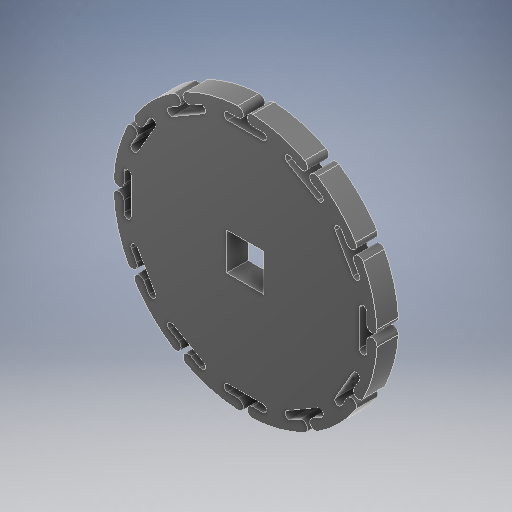
# Autodesk Inventor part: Sprocket
Saved by Autodesk Inventor 2026.1 (Build 301233000, 233)
## iProperties
Created: 2025-10-04
Part Number: Sprocket
Material: Plastic, Opaque Black
Document SubType Name: Modeling
Designer: Teddy
Density: 0.952 g/cm^3
Appearance: Smooth - Black
Author: Teddy
Autodesk Inventor part; units mm, degrees
ref_plane "YZ Plane" through (0, 0, 0) normal (1, 0, 0) x (0, 1, 0)
ref_plane "XZ Plane" through (0, 0, 0) normal (0, 1, 0) x (-1, 0, 0)
ref_plane "XY Plane" through (0, 0, 0) normal (0, 0, 1) x (1, 0, 0)
sketch "Sketch1" plane through (0, 0, 0) normal (0, 0, 1) x (1, 0, 0)
  arc A0 (-1.3226, 23.4577) -> (-10.5835, 20.9763) centre (0, 0) ccw
  line L0 (-3.302, -3.302) -> (3.302, -3.302)
  line L1 (3.302, -3.302) -> (3.302, 3.302)
  line L2 (3.302, 3.302) -> (-3.302, 3.302)
  line L3 (-3.302, 3.302) -> (-3.302, -3.302)
  line L4 (-3.302, -3.302) -> (3.302, 3.302) construction
  line L5 (3.302, -3.302) -> (-3.302, 3.302) construction
  line L6 (0, 0) -> (0, 9.525) construction
  line L7 (-3.175, 20.955) -> (3.175, 20.955)
  line L8 (-3.175, 20.32) -> (3.175, 20.32)
  arc A1 (-3.175, 21.59) -> (-3.175, 20.32) centre (-3.175, 20.955) ccw
  arc A2 (3.175, 20.32) -> (3.175, 21.59) centre (3.175, 20.955) ccw
  arc A3 (-1.27, 21.59) -> (-1.3226, 23.4577) centre (-1.27, 22.5246) ccw
  arc A4 (1.3226, 23.4577) -> (1.27, 21.59) centre (1.27, 22.5246) ccw
  line L9 (-1.27, 22.5246) -> (1.27, 22.5246) construction
  line L10 (3.175, 21.59) -> (1.27, 21.59)
  line L11 (-1.27, 21.59) -> (-3.175, 21.59)
  arc A5 (-13.5446, 17.11) -> (-12.9096, 16.0101) centre (-13.2271, 16.5601) ccw
  line L12 (-12.9096, 16.0101) -> (-7.4104, 19.1851)
  arc A6 (-7.4104, 19.1851) -> (-8.0454, 20.285) centre (-7.7279, 19.7351) ccw
  arc A7 (-10.5835, 20.9763) -> (-9.6951, 19.3325) centre (-10.1625, 20.1419) ccw
  line L13 (-8.0454, 20.285) -> (-9.6951, 19.3325)
  line L14 (-11.8949, 18.0625) -> (-13.5446, 17.11)
  arc A8 (-11.8949, 18.0625) -> (-12.8743, 19.6537) centre (-12.3622, 18.8719) ccw
  arc A9 (-20.285, 8.0454) -> (-19.1851, 7.4104) centre (-19.7351, 7.7279) ccw
  line L15 (-19.1851, 7.4104) -> (-16.0101, 12.9096)
  arc A10 (-16.0101, 12.9096) -> (-17.11, 13.5446) centre (-16.5601, 13.2271) ccw
  arc A11 (-19.6537, 12.8743) -> (-18.0625, 11.8949) centre (-18.8719, 12.3622) ccw
  line L16 (-17.11, 13.5446) -> (-18.0625, 11.8949)
  line L17 (-19.3325, 9.6951) -> (-20.285, 8.0454)
  arc A12 (-19.3325, 9.6951) -> (-20.9763, 10.5835) centre (-20.1419, 10.1625) ccw
  arc A13 (-21.59, -3.175) -> (-20.32, -3.175) centre (-20.955, -3.175) ccw
  line L18 (-20.32, -3.175) -> (-20.32, 3.175)
  arc A14 (-20.32, 3.175) -> (-21.59, 3.175) centre (-20.955, 3.175) ccw
  arc A15 (-23.4577, 1.3226) -> (-21.59, 1.27) centre (-22.5246, 1.27) ccw
  line L19 (-21.59, 3.175) -> (-21.59, 1.27)
  line L20 (-21.59, -1.27) -> (-21.59, -3.175)
  arc A16 (-21.59, -1.27) -> (-23.4577, -1.3226) centre (-22.5246, -1.27) ccw
  arc A17 (-17.11, -13.5446) -> (-16.0101, -12.9096) centre (-16.5601, -13.2271) ccw
  line L21 (-16.0101, -12.9096) -> (-19.1851, -7.4104)
  arc A18 (-19.1851, -7.4104) -> (-20.285, -8.0454) centre (-19.7351, -7.7279) ccw
  arc A19 (-20.9763, -10.5835) -> (-19.3325, -9.6951) centre (-20.1419, -10.1625) ccw
  line L22 (-20.285, -8.0454) -> (-19.3325, -9.6951)
  line L23 (-18.0625, -11.8949) -> (-17.11, -13.5446)
  arc A20 (-18.0625, -11.8949) -> (-19.6537, -12.8743) centre (-18.8719, -12.3622) ccw
  arc A21 (-8.0454, -20.285) -> (-7.4104, -19.1851) centre (-7.7279, -19.7351) ccw
  line L24 (-7.4104, -19.1851) -> (-12.9096, -16.0101)
  arc A22 (-12.9096, -16.0101) -> (-13.5446, -17.11) centre (-13.2271, -16.5601) ccw
  arc A23 (-12.8743, -19.6537) -> (-11.8949, -18.0625) centre (-12.3622, -18.8719) ccw
  line L25 (-13.5446, -17.11) -> (-11.8949, -18.0625)
  line L26 (-9.6951, -19.3325) -> (-8.0454, -20.285)
  arc A24 (-9.6951, -19.3325) -> (-10.5835, -20.9763) centre (-10.1625, -20.1419) ccw
  arc A25 (3.175, -21.59) -> (3.175, -20.32) centre (3.175, -20.955) ccw
  line L27 (3.175, -20.32) -> (-3.175, -20.32)
  arc A26 (-3.175, -20.32) -> (-3.175, -21.59) centre (-3.175, -20.955) ccw
  arc A27 (-1.3226, -23.4577) -> (-1.27, -21.59) centre (-1.27, -22.5246) ccw
  line L28 (-3.175, -21.59) -> (-1.27, -21.59)
  line L29 (1.27, -21.59) -> (3.175, -21.59)
  arc A28 (1.27, -21.59) -> (1.3226, -23.4577) centre (1.27, -22.5246) ccw
  arc A29 (13.5446, -17.11) -> (12.9096, -16.0101) centre (13.2271, -16.5601) ccw
  line L30 (12.9096, -16.0101) -> (7.4104, -19.1851)
  arc A30 (7.4104, -19.1851) -> (8.0454, -20.285) centre (7.7279, -19.7351) ccw
  arc A31 (10.5835, -20.9763) -> (9.6951, -19.3325) centre (10.1625, -20.1419) ccw
  line L31 (8.0454, -20.285) -> (9.6951, -19.3325)
  line L32 (11.8949, -18.0625) -> (13.5446, -17.11)
  arc A32 (11.8949, -18.0625) -> (12.8743, -19.6537) centre (12.3622, -18.8719) ccw
  arc A33 (20.285, -8.0454) -> (19.1851, -7.4104) centre (19.7351, -7.7279) ccw
  line L33 (19.1851, -7.4104) -> (16.0101, -12.9096)
  arc A34 (16.0101, -12.9096) -> (17.11, -13.5446) centre (16.5601, -13.2271) ccw
  arc A35 (19.6537, -12.8743) -> (18.0625, -11.8949) centre (18.8719, -12.3622) ccw
  line L34 (17.11, -13.5446) -> (18.0625, -11.8949)
  line L35 (19.3325, -9.6951) -> (20.285, -8.0454)
  arc A36 (19.3325, -9.6951) -> (20.9763, -10.5835) centre (20.1419, -10.1625) ccw
  arc A37 (21.59, 3.175) -> (20.32, 3.175) centre (20.955, 3.175) ccw
  line L36 (20.32, 3.175) -> (20.32, -3.175)
  arc A38 (20.32, -3.175) -> (21.59, -3.175) centre (20.955, -3.175) ccw
  arc A39 (23.4577, -1.3226) -> (21.59, -1.27) centre (22.5246, -1.27) ccw
  line L37 (21.59, -3.175) -> (21.59, -1.27)
  line L38 (21.59, 1.27) -> (21.59, 3.175)
  arc A40 (21.59, 1.27) -> (23.4577, 1.3226) centre (22.5246, 1.27) ccw
  arc A41 (17.11, 13.5446) -> (16.0101, 12.9096) centre (16.5601, 13.2271) ccw
  line L39 (16.0101, 12.9096) -> (19.1851, 7.4104)
  arc A42 (19.1851, 7.4104) -> (20.285, 8.0454) centre (19.7351, 7.7279) ccw
  arc A43 (20.9763, 10.5835) -> (19.3325, 9.6951) centre (20.1419, 10.1625) ccw
  line L40 (20.285, 8.0454) -> (19.3325, 9.6951)
  line L41 (18.0625, 11.8949) -> (17.11, 13.5446)
  arc A44 (18.0625, 11.8949) -> (19.6537, 12.8743) centre (18.8719, 12.3622) ccw
  arc A45 (8.0454, 20.285) -> (7.4104, 19.1851) centre (7.7279, 19.7351) ccw
  line L42 (7.4104, 19.1851) -> (12.9096, 16.0101)
  arc A46 (12.9096, 16.0101) -> (13.5446, 17.11) centre (13.2271, 16.5601) ccw
  arc A47 (12.8743, 19.6537) -> (11.8949, 18.0625) centre (12.3622, 18.8719) ccw
  line L43 (13.5446, 17.11) -> (11.8949, 18.0625)
  line L44 (9.6951, 19.3325) -> (8.0454, 20.285)
  arc A48 (9.6951, 19.3325) -> (10.5835, 20.9763) centre (10.1625, 20.1419) ccw
  arc A49 (-12.8743, 19.6537) -> (-19.6537, 12.8743) centre (0, 0) ccw
  arc A50 (-10.5835, 20.9763) -> (-12.8743, 19.6537) centre (0, 0) ccw construction
  arc A51 (10.5835, 20.9763) -> (1.3226, 23.4577) centre (0, 0) ccw
  arc A52 (12.8743, 19.6537) -> (10.5835, 20.9763) centre (0, 0) ccw construction
  arc A53 (19.6537, 12.8743) -> (12.8743, 19.6537) centre (0, 0) ccw
  arc A54 (20.9763, 10.5835) -> (19.6537, 12.8743) centre (0, 0) ccw construction
  arc A55 (23.4577, 1.3226) -> (20.9763, 10.5835) centre (0, 0) ccw
  arc A56 (23.4577, -1.3226) -> (23.4577, 1.3226) centre (0, 0) ccw construction
  arc A57 (20.9763, -10.5835) -> (23.4577, -1.3226) centre (0, 0) ccw
  arc A58 (19.6537, -12.8743) -> (20.9763, -10.5835) centre (0, 0) ccw construction
  arc A59 (12.8743, -19.6537) -> (19.6537, -12.8743) centre (0, 0) ccw
  arc A60 (10.5835, -20.9763) -> (12.8743, -19.6537) centre (0, 0) ccw construction
  arc A61 (1.3226, -23.4577) -> (10.5835, -20.9763) centre (0, 0) ccw
  arc A62 (-1.3226, -23.4577) -> (1.3226, -23.4577) centre (0, 0) ccw construction
  arc A63 (-12.8743, -19.6537) -> (-10.5835, -20.9763) centre (0, 0) ccw construction
  arc A64 (-10.5835, -20.9763) -> (-1.3226, -23.4577) centre (0, 0) ccw
  arc A65 (-20.9763, -10.5835) -> (-19.6537, -12.8743) centre (0, 0) ccw construction
  arc A66 (-19.6537, -12.8743) -> (-12.8743, -19.6537) centre (0, 0) ccw
  arc A67 (-23.4577, -1.3226) -> (-20.9763, -10.5835) centre (0, 0) ccw
  arc A68 (-23.4577, 1.3226) -> (-23.4577, -1.3226) centre (0, 0) ccw construction
  arc A69 (-19.6537, 12.8743) -> (-20.9763, 10.5835) centre (0, 0) ccw construction
  arc A70 (-20.9763, 10.5835) -> (-23.4577, 1.3226) centre (0, 0) ccw
  point P0 (0, 20.955)
  dimension "d0" = 46.99
  dimension "d1" = 6.604
  dimension "d2" = 6.604
  dimension "d3" = 20.955
  dimension "d4" = 6.35
  dimension "d5" = 2.54
  dimension "d6" = 0.635
  dimension "d11" = 360
  constraints: 96 point on circle, 90 end point, 48 centre point, 48 equal radius, 36 equal length, 10 tangent, 4 horizontal, 4 parallel, 3 vertical alignment, 2 horizontal alignment, 2 perpendicular, 1 midpoint, 217 other
  measures "d1" distance of L2.end L1.end
  measures "d2" distance of L0.end L1.end
  measures "d3" distance from line of point (0, 0) L7
  measures "d4" distance of L7.start L7.end
  measures "d5" distance of L9.start L9.end
  measures "d6" distance between parallel lines of L7 L8
extrude "Extrusion1" add sketch "Sketch1" along normal blind 3.81
body "Solid1"
